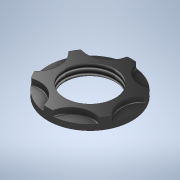
# Autodesk Inventor part: Part2
Saved by Autodesk Inventor 2020 (Build 240168000, 168)
## iProperties
Created: 2021-05-18
Part Number: Part2
Material: Steel, Alloy
Document SubType Name: Modeling
Designer: Andrew
Density: 7.73 g/cm^3
Appearance: Glossy - Black
Mass: 170.874 g
Surface Area: 94.2017 cm^2
Volume: 22.1053 cm^3
Author: Andrew
Autodesk Inventor part; units mm, degrees
ref_plane "YZ Plane" through (0, 0, 0) normal (1, 0, 0) x (0, 1, 0)
ref_plane "XZ Plane" through (0, 0, 0) normal (0, 1, 0) x (-1, 0, 0)
ref_plane "XY Plane" through (0, 0, 0) normal (0, 0, 1) x (1, 0, 0)
sketch "Sketch1" plane through (0, 0, 0) normal (0, 1, 0) x (-1, 0, 0)
  circle A0 centre (0, 0) radius 22.5
  circle A1 centre (0, 0) radius 37.5
  circle A2 centre (47.5, 0) radius 20
  point P0 (34.3421, -15.0622)
  point P1 (34.3421, 15.0622)
  dimension "d0" = 45
  dimension "d1" = 75
  dimension "d2" = 40
  dimension "d3" = 47.5
  constraints: 3 centre point, 2 coincident
  measures "d0" diameter of A0
  measures "d1" diameter of A1
  measures "d2" diameter of A2
  measures "d3" distance of A2.centre point (0, 0)
extrude "Extrusion1" add sketch "Sketch1" against normal blind 10 contours A1 A2 | A2 A1 picked at (34.0976, 2.5269) picked at (-32.1783, -2.8175)
extrude "Extrusion2" cut sketch "Sketch1" against normal blind 5 contours A1 A2 picked at (34.0976, 2.5269)
pattern_circular "Circular Pattern1" count 6 over 360 about axis through (0, 0, 0) along (0, -1, 0) of "Extrusion2"
fillet "Fillet1" radius 1 18 edges at (-34.3421, -2.5, -15.0622) (-34.3421, -2.5, 15.0622) (-27.5, -5, 0) (-30.2153, -2.5, 22.21) (-4.1268, -2.5, 37.2722) (-13.75, -5, 23.8157) (4.1268, -2.5, 37.2722) (30.2153, -2.5, 22.21) (13.75, -5, 23.8157) (-4.1268, -2.5, -37.2722) (-30.2153, -2.5, -22.21) (-13.75, -5, -23.8157) (30.2153, -2.5, -22.21) (4.1268, -2.5, -37.2722) (13.75, -5, -23.8157) (34.3421, -2.5, 15.0622) (34.3421, -2.5, -15.0622) (27.5, -5, 0)
thread "Thread1" size "M45x4.5" class "6H" standard "ANSI Metric M Profile" length 10
body "Solid1"
